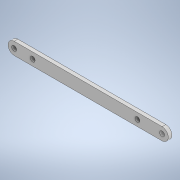
# Autodesk Inventor part: 零件2
Saved by Autodesk Inventor 2022 (Build 260153000, 153)
## iProperties
Created: 2023-04-16
Part Number: 零件2
Material: 一般
Document SubType Name: Modeling
Designer: JOU
Density: 1 g/cm^3
Appearance: 預設
Author: JOU
Autodesk Inventor part; units mm, degrees
ref_plane "YZ Plane" through (0, 0, 0) normal (1, 0, 0) x (0, 1, 0)
ref_plane "XZ Plane" through (0, 0, 0) normal (0, 1, 0) x (-1, 0, 0)
ref_plane "XY Plane" through (0, 0, 0) normal (0, 0, 1) x (1, 0, 0)
sketch "草圖1" plane through (0, 0, 0) normal (0, 0, 1) x (1, 0, 0)
  line L0 (-223.1596, 56.676) -> (-103.1596, 56.676) construction
  line L1 (-223.1596, 51.676) -> (-103.1596, 51.676)
  line L2 (-103.1596, 61.676) -> (-223.1596, 61.676)
  arc A0 (-223.1596, 61.676) -> (-223.1596, 51.676) centre (-223.1596, 56.676) ccw
  arc A1 (-103.1596, 51.676) -> (-103.1596, 61.676) centre (-103.1596, 56.676) ccw
  circle A2 centre (-223.1596, 56.676) radius 2
  circle A3 centre (-103.1596, 56.676) radius 2
  circle A4 centre (-208.1596, 56.676) radius 2
  circle A5 centre (-123.1596, 56.676) radius 2
  point P0 (0, 0)
  point P1 (-163.1596, 56.676)
  dimension "d0" = 120
  dimension "d1" = 10
  dimension "d2" = 4
  dimension "d3" = 4
  dimension "d4" = 4
  dimension "d5" = 15
  dimension "d8" = 4
  dimension "d9" = 20
  constraints: 8 end point, 6 centre point, 4 point on circle, 4 tangent, 2 coincident, 2 point on line, 1 horizontal, 1 midpoint, 1 parallel
  measures "d0" distance of L2.start L2.end
  measures "d1" distance between parallel lines of L1 L2
  measures "d2" diameter of A2
  measures "d3" diameter of A3
  measures "d4" diameter of A4
  measures "d5" distance of A4.centre A2.centre
  measures "d8" diameter of A5
  measures "d9" distance of L0.end A5.centre
extrude "擠出1" add sketch "草圖1" along normal blind 3
